Autodesk Inventor part; units mm, degrees
(part 2 of 2)
  spline S173 degree 2 poles (16.9034, -201.3098) (17.5444, -201.3098) (18.2669, -201.9878) (18.2669, -202.5658) knots 0 0 0 1 2 2 2
  spline S174 degree 2 poles (18.2669, -202.5658) (18.2669, -202.8363) (18.1409, -203.2883) (18.0297, -203.481) knots 0 0 0 1 2 2 2
  spline S175 degree 2 poles (18.0297, -203.481) (17.9186, -203.681) (17.5963, -204.0738) (17.4184, -204.2627) knots 0 0 0 1 2 2 2
  spline S176 degree 2 poles (17.4184, -204.2627) (17.1294, -204.5777) (16.4218, -205.252) (16.2106, -205.4483) knots 0 0 0 1 2 2 2
  line L141 (16.2106, -205.4483) -> (18.4558, -205.4483)
  line L142 (18.4558, -205.4483) -> (18.4558, -205.9782)
  line L143 (20.9678, -201.2024) -> (19.1783, -206.9711)
  line L144 (19.1783, -206.9711) -> (18.6596, -206.9711)
  line L145 (18.6596, -206.9711) -> (20.4417, -201.2024)
  line L146 (20.4417, -201.2024) -> (20.9678, -201.2024)
  line L147 (24.2912, -205.9782) -> (21.4717, -205.9782)
  line L148 (21.4717, -205.9782) -> (21.4717, -205.3298)
  spline S177 degree 2 poles (21.4717, -205.3298) (21.7755, -205.0445) (22.3165, -204.5147) (22.5758, -204.2294) knots 0 0 0 1 2 2 2
  spline S178 degree 2 poles (22.5758, -204.2294) (23.0982, -203.6551) (23.4798, -202.966) (23.4798, -202.5992) knots 0 0 0 1 2 2 2
  spline S179 degree 2 poles (23.4798, -202.5992) (23.4798, -202.4065) (23.3613, -202.1175) (23.2538, -202.0249) knots 0 0 0 1 2 2 2
  spline S180 degree 2 poles (23.2538, -202.0249) (23.1464, -201.9323) (22.8648, -201.8396) (22.6944, -201.8396) knots 0 0 0 1 2 2 2
  spline S181 degree 2 poles (22.6944, -201.8396) (22.5314, -201.8396) (22.1979, -201.9211) (22.046, -201.9841) knots 0 0 0 1 2 2 2
  spline S182 degree 2 poles (22.046, -201.9841) (21.9163, -202.036) (21.6755, -202.1842) (21.6014, -202.2361) knots 0 0 0 1 2 2 2
  line L149 (21.6014, -202.2361) -> (21.568, -202.2361)
  line L150 (21.568, -202.2361) -> (21.568, -201.584)
  spline S183 degree 2 poles (21.568, -201.584) (21.757, -201.4914) (22.435, -201.3098) (22.7388, -201.3098) knots 0 0 0 1 2 2 2
  spline S184 degree 2 poles (22.7388, -201.3098) (23.3798, -201.3098) (24.1023, -201.9878) (24.1023, -202.5658) knots 0 0 0 1 2 2 2
  spline S185 degree 2 poles (24.1023, -202.5658) (24.1023, -202.8363) (23.9763, -203.2883) (23.8652, -203.481) knots 0 0 0 1 2 2 2
  spline S186 degree 2 poles (23.8652, -203.481) (23.754, -203.681) (23.4317, -204.0738) (23.2538, -204.2627) knots 0 0 0 1 2 2 2
  spline S187 degree 2 poles (23.2538, -204.2627) (22.9648, -204.5777) (22.2572, -205.252) (22.046, -205.4483) knots 0 0 0 1 2 2 2
  line L151 (22.046, -205.4483) -> (24.2912, -205.4483)
  line L152 (24.2912, -205.4483) -> (24.2912, -205.9782)
  spline S188 degree 2 poles (27.748, -203.6922) (27.748, -204.9222) (27.033, -206.0745) (26.2882, -206.0745) knots 0 0 0 1 2 2 2
  spline S189 degree 2 poles (26.2882, -206.0745) (25.5324, -206.0745) (24.8248, -204.9) (24.8248, -203.6959) knots 0 0 0 1 2 2 2
  spline S190 degree 2 poles (24.8248, -203.6959) (24.8248, -202.4584) (25.5398, -201.3135) (26.2882, -201.3135) knots 0 0 0 1 2 2 2
  spline S191 degree 2 poles (26.2882, -201.3135) (27.0404, -201.3135) (27.748, -202.4991) (27.748, -203.6922) knots 0 0 0 1 2 2 2
  spline S192 degree 2 poles (26.9626, -205.0852) (27.0515, -204.8592) (27.1256, -204.1627) (27.1256, -203.6922) knots 0 0 0 1 2 2 2
  spline S193 degree 2 poles (27.1256, -203.6922) (27.1256, -203.2216) (27.0515, -202.5288) (26.9589, -202.2954) knots 0 0 0 1 2 2 2
  spline S194 degree 2 poles (26.9589, -202.2954) (26.8662, -202.0619) (26.5439, -201.8211) (26.2882, -201.8211) knots 0 0 0 1 2 2 2
  spline S195 degree 2 poles (26.2882, -201.8211) (26.0326, -201.8211) (25.7029, -202.0619) (25.6065, -202.3028) knots 0 0 0 1 2 2 2
  spline S196 degree 2 poles (25.6065, -202.3028) (25.5139, -202.5362) (25.4472, -203.2475) (25.4472, -203.6959) knots 0 0 0 1 2 2 2
  spline S197 degree 2 poles (25.4472, -203.6959) (25.4472, -204.1775) (25.5065, -204.8222) (25.6028, -205.0741) knots 0 0 0 1 2 2 2
  spline S198 degree 2 poles (25.6028, -205.0741) (25.6917, -205.3112) (26.0215, -205.5669) (26.2882, -205.5669) knots 0 0 0 1 2 2 2
  spline S199 degree 2 poles (26.2882, -205.5669) (26.5402, -205.5669) (26.8699, -205.3261) (26.9626, -205.0852) knots 0 0 0 1 2 2 2
  line L153 (31.1529, -205.9782) -> (28.3334, -205.9782)
  line L154 (28.3334, -205.9782) -> (28.3334, -205.3298)
  spline S200 degree 2 poles (28.3334, -205.3298) (28.6372, -205.0445) (29.1782, -204.5147) (29.4375, -204.2294) knots 0 0 0 1 2 2 2
  spline S201 degree 2 poles (29.4375, -204.2294) (29.9599, -203.6551) (30.3415, -202.966) (30.3415, -202.5992) knots 0 0 0 1 2 2 2
  spline S202 degree 2 poles (30.3415, -202.5992) (30.3415, -202.4065) (30.223, -202.1175) (30.1155, -202.0249) knots 0 0 0 1 2 2 2
  spline S203 degree 2 poles (30.1155, -202.0249) (30.0081, -201.9323) (29.7265, -201.8396) (29.5561, -201.8396) knots 0 0 0 1 2 2 2
  spline S204 degree 2 poles (29.5561, -201.8396) (29.3931, -201.8396) (29.0596, -201.9211) (28.9077, -201.9841) knots 0 0 0 1 2 2 2
  spline S205 degree 2 poles (28.9077, -201.9841) (28.778, -202.036) (28.5372, -202.1842) (28.4631, -202.2361) knots 0 0 0 1 2 2 2
  line L155 (28.4631, -202.2361) -> (28.4297, -202.2361)
  line L156 (28.4297, -202.2361) -> (28.4297, -201.584)
  spline S206 degree 2 poles (28.4297, -201.584) (28.6187, -201.4914) (29.2967, -201.3098) (29.6005, -201.3098) knots 0 0 0 1 2 2 2
  spline S207 degree 2 poles (29.6005, -201.3098) (30.2415, -201.3098) (30.964, -201.9878) (30.964, -202.5658) knots 0 0 0 1 2 2 2
  spline S208 degree 2 poles (30.964, -202.5658) (30.964, -202.8363) (30.838, -203.2883) (30.7269, -203.481) knots 0 0 0 1 2 2 2
  spline S209 degree 2 poles (30.7269, -203.481) (30.6157, -203.681) (30.2934, -204.0738) (30.1155, -204.2627) knots 0 0 0 1 2 2 2
  spline S210 degree 2 poles (30.1155, -204.2627) (29.8265, -204.5777) (29.1189, -205.252) (28.9077, -205.4483) knots 0 0 0 1 2 2 2
  line L157 (28.9077, -205.4483) -> (31.1529, -205.4483)
  line L158 (31.1529, -205.4483) -> (31.1529, -205.9782)
  spline S211 degree 2 poles (34.6542, -204.4961) (34.6542, -204.8481) (34.4208, -205.4446) (34.2244, -205.6447) knots 0 0 0 1 2 2 2
  spline S212 degree 2 poles (34.2244, -205.6447) (34.0206, -205.8559) (33.5093, -206.0745) (33.2018, -206.0745) knots 0 0 0 1 2 2 2
  spline S213 degree 2 poles (33.2018, -206.0745) (32.8943, -206.0745) (32.3867, -205.867) (32.1941, -205.6595) knots 0 0 0 1 2 2 2
  spline S214 degree 2 poles (32.1941, -205.6595) (31.9569, -205.4113) (31.6902, -204.5777) (31.6902, -203.97) knots 0 0 0 1 2 2 2
  spline S215 degree 2 poles (31.6902, -203.97) (31.6902, -203.3735) (31.9347, -202.4139) (32.1903, -202.0582) knots 0 0 0 1 2 2 2
  spline S216 degree 2 poles (32.1903, -202.0582) (32.4386, -201.71) (33.2241, -201.3209) (33.739, -201.3209) knots 0 0 0 1 2 2 2
  spline S217 degree 2 poles (33.739, -201.3209) (33.891, -201.3209) (34.1577, -201.3506) (34.2578, -201.3839) knots 0 0 0 1 2 2 2
  line L159 (34.2578, -201.3839) -> (34.2578, -201.973)
  line L160 (34.2578, -201.973) -> (34.2318, -201.973)
  spline S218 degree 2 poles (34.2318, -201.973) (34.1466, -201.9286) (33.8354, -201.8508) (33.6575, -201.8508) knots 0 0 0 1 2 2 2
  spline S219 degree 2 poles (33.6575, -201.8508) (33.087, -201.8508) (32.3867, -202.6214) (32.32, -203.3772) knots 0 0 0 1 2 2 2
  spline S220 degree 2 poles (32.32, -203.3772) (32.5386, -203.2253) (32.998, -203.0586) (33.2722, -203.0586) knots 0 0 0 1 2 2 2
  spline S221 degree 2 poles (33.2722, -203.0586) (33.539, -203.0586) (33.9391, -203.166) (34.1577, -203.3291) knots 0 0 0 1 2 2 2
  spline S222 degree 2 poles (34.1577, -203.3291) (34.4097, -203.518) (34.6542, -204.1034) (34.6542, -204.4961) knots 0 0 0 1 2 2 2
  spline S223 degree 2 poles (34.0317, -204.5221) (34.0317, -204.2405) (33.8835, -203.8589) (33.7205, -203.7255) knots 0 0 0 1 2 2 2
  spline S224 degree 2 poles (33.7205, -203.7255) (33.5983, -203.6292) (33.2944, -203.5662) (33.1351, -203.5662) knots 0 0 0 1 2 2 2
  spline S225 degree 2 poles (33.1351, -203.5662) (32.9202, -203.5662) (32.5164, -203.6959) (32.32, -203.8181) knots 0 0 0 1 2 2 2
  spline S226 degree 2 poles (32.32, -203.8181) (32.3163, -203.8848) (32.3089, -204.0108) (32.3089, -204.1071) knots 0 0 0 1 2 2 2
  spline S227 degree 2 poles (32.3089, -204.1071) (32.3089, -204.5814) (32.4942, -205.163) (32.635, -205.315) knots 0 0 0 1 2 2 2
  spline S228 degree 2 poles (32.635, -205.315) (32.7646, -205.4594) (33.0462, -205.5743) (33.2055, -205.5743) knots 0 0 0 1 2 2 2
  spline S229 degree 2 poles (33.2055, -205.5743) (33.576, -205.5743) (34.0317, -205.0482) (34.0317, -204.5221) knots 0 0 0 1 2 2 2
  point P0 (0, 0)
  constraints: 2 other
emboss "Emboss1" sketch "Sketch14" operation cut depth 2.54 direction (-1, 0, 0)
sketch "Sketch16" plane through (5.08, 0, 0) normal (1, 0, 0) x (0, 0, -1)
  line L0 (-45.5467, -73.9362) -> (38.2733, -73.9362)
  line L1 (38.2733, -73.9362) -> (38.2733, -77.7462)
  line L2 (38.2733, -77.7462) -> (-45.5467, -77.7462)
  line L3 (-45.5467, -77.7462) -> (-45.5467, -73.9362)
  line L4 (38.9083, -211.0962) -> (-46.1817, -211.0962) projected
  line L5 (42.0833, 28.0448) -> (42.0833, -207.9212) projected
  line L6 (-49.3567, -207.9212) -> (-49.3567, 28.0448) projected
  point P0 (0, 0)
  point P1 (38.9083, -223.7962)
  point P2 (42.0833, -220.6212)
  point P3 (38.2733, -75.8412)
  point P4 (-45.5467, -75.8412)
  dimension "d195" = 3.81
  dimension "d692" = 137.16
  dimension "d796" = 3.81
  dimension "d797" = 3.81
  constraints: 8 end point, 2 midpoint, 2 parallel, 1 horizontal, 1 perpendicular, 1 other
  measures "d195" distance between parallel lines of L0 L2
  measures "d796" distance from line of L5 point (38.273, -75.841)
  measures "d797" distance from line of L6 point (-45.547, -75.841)
extrude "Extrusion13" add sketch "Sketch16" along normal blind 5.08
sketch "Sketch17" plane through (24.13, 33.2264, 43.0067) normal (0, 1, 0) x (1, 0, 0)
  line L0 (-8.128, 57.15) -> (0, 57.15) projected
  line L1 (-0.0061, 57.15) -> (0.0392, 57.15)
  line L2 (0, 87.0966) -> (0, -8.3566) projected
  line L3 (0, 35.5801) -> (0, 35.5243)
  line L4 (5, -5.1816) -> (5, 83.9216) projected
  line L5 (0, 57.15) -> (5, 57.15)
  line L6 (5, 57.15) -> (5, 0)
  line L7 (5, 0) -> (0, 0)
  line L8 (0, 0) -> (0, 57.15)
  line L9 (0, 0) -> (-8.128, 0) projected
  point P0 (-24.13, 43.0067)
  point P1 (5, -23.8506)
  point P2 (5, 69.0626)
  point P3 (0, 0)
  point P4 (5, 57.15)
  point P5 (2.5, 0)
  point P6 (2.5, 57.15)
  dimension "d689" = 57.15
  dimension "d1196" = 0
  constraints: 12 end point, 4 point on line, 2 horizontal, 2 midpoint, 2 parallel, 1 perpendicular
  measures "d689" distance of point (2.5, 0) point (2.5, 57.15)
  measures "d1196" distance between parallel lines of L7 L9
extrude "Extrusion14" cut sketch "Sketch17" against normal blind 2.0066
sketch "Sketch18" plane through (0, 0, 0) normal (-1, 0, 0) x (0, 0, 1)
  arc A0 (48.3408, 33.2227) -> (51.3596, 30.2039) centre (50.6267, 32.4898) ccw projected
  circle A1 centre (50.6267, 32.4898) radius 4.5085
  arc A2 (-41.0674, 33.2227) -> (-44.0862, 30.2039) centre (-43.3533, 32.4898) ccw projected
  circle A3 centre (-43.3533, 32.4898) radius 4.5085
  arc A4 (-44.0862, -210.0804) -> (-41.0674, -213.0992) centre (-43.3533, -212.3662) ccw projected
  circle A5 centre (-43.3533, -212.3662) radius 4.5085
  arc A6 (48.3408, -213.0992) -> (51.3596, -210.0804) centre (50.6267, -212.3662) ccw projected
  circle A7 centre (50.6267, -212.3662) radius 4.5085
  point P0 (0, 0)
  point P1 (-44.0899, -210.0815)
  point P2 (-44.0899, -214.6509)
  point P3 (48.8233, -214.6509)
  point P4 (48.8233, -210.0815)
  point P5 (-41.0686, 33.2264)
  point P6 (-41.0686, -213.1028)
  dimension "d209" = 9.017
  dimension "d210" = 9.017
  dimension "d211" = 9.017
  dimension "d212" = 9.017
  constraints: 4 centre point, 4 coincident
  measures "d209" diameter of A1
  measures "d210" diameter of A3
  measures "d211" diameter of A5
  measures "d212" diameter of A7
extrude "Extrusion15" [suppressed]
sketch "Sketch19" plane through (24.13, -51.5842, -44.0899) normal (0, 0, -1) x (-1, 0, 0)
  line L0 (7.62, 0) -> (0, 0) projected
  line L1 (-5, 79.629) -> (-5, -156.337) projected
  line L2 (0, 0) -> (-5, 0)
  line L3 (-5, 0) -> (-5, 8.001)
  line L4 (-5, 8.001) -> (0, 8.001)
  line L5 (0, 8.001) -> (0, 0)
  point P0 (24.13, 51.5842)
  point P1 (-5, -156.337)
  dimension "d216" = 5
  dimension "d219" = 8.001
  constraints: 8 end point, 2 parallel, 1 horizontal, 1 perpendicular, 1 point on line
  measures "d216" distance between parallel lines of L1 L5
  measures "d219" distance between parallel lines of L2 L4
extrude "Extrusion16" cut sketch "Sketch19" against normal blind 24.13
sketch "Sketch20" plane through (0, 0, 0) normal (-1, 0, 0) x (0, 0, 1)
  line L0 (-45.1249, 28.9592) -> (-41.5943, 28.9592)
  line L1 (-45.1249, 36.0204) -> (-41.5943, 36.0204)
  line L2 (-45.1249, 28.9592) -> (-47.1633, 32.4898)
  line L3 (-45.1249, 36.0204) -> (-47.1633, 32.4898)
  line L4 (-41.5943, 28.9592) -> (-39.5559, 32.4898)
  line L5 (-41.5943, 36.0204) -> (-39.5559, 32.4898)
  line L6 (-45.1249, -215.8968) -> (-41.5943, -215.8968)
  line L7 (-45.1249, -208.8356) -> (-41.5943, -208.8356)
  line L8 (-45.1249, -215.8968) -> (-47.1633, -212.3662)
  line L9 (-45.1249, -208.8356) -> (-47.1633, -212.3662)
  line L10 (-41.5943, -215.8968) -> (-39.5559, -212.3662)
  line L11 (-41.5943, -208.8356) -> (-39.5559, -212.3662)
  line L12 (48.8551, 28.9592) -> (52.3857, 28.9592)
  line L13 (48.8551, 36.0204) -> (52.3857, 36.0204)
  line L14 (48.8551, 28.9592) -> (46.8167, 32.4898)
  line L15 (48.8551, 36.0204) -> (46.8167, 32.4898)
  line L16 (52.3857, 28.9592) -> (54.4241, 32.4898)
  line L17 (52.3857, 36.0204) -> (54.4241, 32.4898)
  line L18 (48.8551, -215.8968) -> (52.3857, -215.8968)
  line L19 (48.8551, -208.8356) -> (52.3857, -208.8356)
  line L20 (48.8551, -215.8968) -> (46.8167, -212.3662)
  line L21 (48.8551, -208.8356) -> (46.8167, -212.3662)
  line L22 (52.3857, -215.8968) -> (54.4241, -212.3662)
  line L23 (52.3857, -208.8356) -> (54.4241, -212.3662)
  line L24 (-40.0449, -67.5608) -> (-36.5143, -67.5608)
  line L25 (-40.0449, -60.4996) -> (-36.5143, -60.4996)
  line L26 (-40.0449, -67.5608) -> (-42.0833, -64.0302)
  line L27 (-40.0449, -60.4996) -> (-42.0833, -64.0302)
  line L28 (-36.5143, -67.5608) -> (-34.4759, -64.0302)
  line L29 (-36.5143, -60.4996) -> (-34.4759, -64.0302)
  line L30 (43.7751, -67.5608) -> (47.3057, -67.5608)
  line L31 (43.7751, -60.4996) -> (47.3057, -60.4996)
  line L32 (43.7751, -67.5608) -> (41.7367, -64.0302)
  line L33 (43.7751, -60.4996) -> (41.7367, -64.0302)
  line L34 (47.3057, -67.5608) -> (49.3441, -64.0302)
  line L35 (47.3057, -60.4996) -> (49.3441, -64.0302)
  point P0 (0, 0)
  point P1 (-16.6833, 31.2198)
  point P2 (-43.3596, 28.9592)
  point P3 (-43.3533, 32.4898)
  point P4 (-43.3596, -215.8968)
  point P5 (50.6204, 28.9592)
  point P6 (50.6204, -215.8968)
  point P7 (-38.2796, -67.5608)
  point P8 (45.5404, -67.5608)
  dimension "d963" = 7.0612
  dimension "d964" = 120
  dimension "d965" = 120
  dimension "d966" = 120
  dimension "d967" = 120
  dimension "d968" = 3.5306
  dimension "d969" = 3.5306
  dimension "d970" = 3.5306
  dimension "d971" = 3.5306
  dimension "d972" = 3.5306
  dimension "d973" = 3.5306
  dimension "d974" = 0
  dimension "d975" = 7.6074
  dimension "d1031" = 7.0612
  dimension "d1032" = 120
  dimension "d1033" = 120
  dimension "d1034" = 120
  dimension "d1035" = 120
  dimension "d1036" = 3.5306
  dimension "d1037" = 3.5306
  dimension "d1038" = 3.5306
  dimension "d1039" = 3.5306
  dimension "d1040" = 3.5306
  dimension "d1041" = 3.5306
  dimension "d1042" = 0
  dimension "d1043" = 7.6074
  dimension "d1082" = 7.0612
  dimension "d1083" = 120
  dimension "d1084" = 120
  dimension "d1085" = 120
  dimension "d1086" = 120
  dimension "d1087" = 3.5306
  dimension "d1088" = 3.5306
  dimension "d1089" = 3.5306
  dimension "d1090" = 3.5306
  dimension "d1091" = 3.5306
  dimension "d1092" = 3.5306
  dimension "d1093" = 0
  dimension "d1094" = 7.6074
  dimension "d1116" = 7.0612
  dimension "d1117" = 120
  dimension "d1118" = 120
  dimension "d1119" = 120
  dimension "d1120" = 120
  dimension "d1121" = 3.5306
  dimension "d1122" = 3.5306
  dimension "d1123" = 3.5306
  dimension "d1124" = 3.5306
  dimension "d1125" = 3.5306
  dimension "d1126" = 3.5306
  dimension "d1127" = 0
  dimension "d1128" = 7.6074
  dimension "d1160" = 7.0612
  dimension "d1161" = 120
  dimension "d1162" = 120
  dimension "d1163" = 120
  dimension "d1164" = 120
  dimension "d1165" = 3.5306
  dimension "d1166" = 3.5306
  dimension "d1167" = 3.5306
  dimension "d1168" = 3.5306
  dimension "d1169" = 3.5306
  dimension "d1170" = 3.5306
  dimension "d1171" = 0
  constraints: 72 end point, 12 horizontal, 6 midpoint
  measures "d963" distance from line of point (-43.36, 28.959) L1
  measures "d964" angle of L0 L2
  measures "d965" angle of L1 L3
  measures "d966" angle of L4 L0
  measures "d967" angle of L5 L1
  measures "d968" distance of L0.start L4.start
  measures "d969" distance of L1.start L5.start
  measures "d970" vertical distance of L1.start L3.end
  measures "d971" vertical distance of L0.start L2.end
  measures "d972" vertical distance of L5.start L5.end
  measures "d973" vertical distance of L4.start L4.end
  measures "d974" horizontal distance of L0.start L1.start
  measures "d975" distance of L4.end L2.end
  measures "d1031" distance from line of point (-43.36, -215.897) L7
  measures "d1032" angle of L6 L8
  measures "d1033" angle of L7 L9
  measures "d1034" angle of L10 L6
  measures "d1035" angle of L11 L7
  measures "d1036" distance of L6.start L10.start
  measures "d1037" distance of L7.start L11.start
  measures "d1038" vertical distance of L7.start L9.end
  measures "d1039" vertical distance of L6.start L8.end
  measures "d1040" vertical distance of L11.start L11.end
  measures "d1041" vertical distance of L10.start L10.end
  measures "d1042" horizontal distance of L6.start L7.start
  measures "d1043" distance of L10.end L8.end
  measures "d1082" distance from line of point (50.62, 28.959) L13
  measures "d1083" angle of L12 L14
  measures "d1084" angle of L13 L15
  measures "d1085" angle of L16 L12
  measures "d1086" angle of L17 L13
  measures "d1087" distance of L12.start L16.start
  measures "d1088" distance of L15.start L17.start
  measures "d1089" vertical distance of L15.start L15.end
  measures "d1090" vertical distance of L12.start L14.end
  measures "d1091" vertical distance of L17.start L17.end
  measures "d1092" vertical distance of L16.start L16.end
  measures "d1093" horizontal distance of L12.start L15.start
  measures "d1094" distance of L16.end L14.end
  measures "d1116" distance from line of point (50.62, -215.897) L19
  measures "d1117" angle of L18 L20
  measures "d1118" angle of L19 L21
  measures "d1119" angle of L22 L18
  measures "d1120" angle of L23 L19
  measures "d1121" distance of L18.start L22.start
  measures "d1122" distance of L21.start L23.start
  measures "d1123" vertical distance of L21.start L21.end
  measures "d1124" vertical distance of L18.start L20.end
  measures "d1125" vertical distance of L23.start L23.end
  measures "d1126" vertical distance of L22.start L22.end
  measures "d1127" horizontal distance of L18.start L21.start
  measures "d1128" distance of L22.end L20.end
  measures "d1160" distance from line of point (-38.28, -67.561) L25
  measures "d1161" angle of L24 L26
  measures "d1162" angle of L25 L27
  measures "d1163" angle of L28 L24
  measures "d1164" angle of L29 L25
  measures "d1165" distance of L24.start L28.start
  measures "d1166" distance of L25.start L29.start
  measures "d1167" vertical distance of L25.start L27.end
  measures "d1168" vertical distance of L24.start L26.end
  measures "d1169" vertical distance of L29.start L29.end
  measures "d1170" vertical distance of L28.start L28.end
  measures "d1171" horizontal distance of L24.start L25.start
extrude "Extrusion18" cut sketch "Sketch20" against normal blind 4
sketch "Sketch21" plane through (5.08, 0, 0) normal (1, 0, 0) x (0, 0, -1)
  line L0 (-49.3567, -207.9212) -> (-49.3567, 28.0448) projected
  line L1 (42.0833, -69.6717) -> (42.0833, -83.8957)
  line L2 (44.0899, -209.9278) -> (44.0899, -51.5842) projected
  line L3 (-49.3567, -83.8422) -> (-49.3567, -69.6182)
  line L4 (-42.4987, -58.8939) -> (-42.4987, -69.23)
  line L5 (-44.2301, -72.0578) -> (-47.3797, -73.6657)
  line L6 (-48.7308, -74.9867) -> (-49.3567, -76.1476)
  line L7 (-44.2301, -56.0661) -> (-47.3797, -54.4582)
  line L8 (-48.7639, -53.074) -> (-49.3567, -51.9128)
  arc A0 (-47.3797, -73.6657) -> (-48.7308, -74.9867) centre (-45.9361, -76.4935) ccw
  arc A1 (-44.2301, -72.0578) -> (-42.4987, -69.23) centre (-45.6737, -69.23) ccw
  arc A2 (-42.4987, -58.8939) -> (-44.2301, -56.0661) centre (-45.6737, -58.8939) ccw
  arc A3 (-48.7639, -53.074) -> (-47.3797, -54.4582) centre (-45.9361, -51.6304) ccw
  line L9 (-49.3567, -51.9128) -> (-49.3567, -76.1476)
  arc A4 (-47.9472, -64.0302) -> (-47.9472, -64.0302) centre (-45.5467, -64.0302) ccw projected
  circle A5 centre (-45.5467, -64.0302) radius 2.4005
  line L10 (35.2253, -69.1835) -> (35.2253, -58.8478)
  line L11 (36.9569, -56.0198) -> (40.1065, -54.4123)
  line L12 (41.4675, -53.0729) -> (42.0833, -51.9128)
  line L13 (36.9569, -72.0115) -> (40.1065, -73.619)
  line L14 (41.4675, -74.9584) -> (42.0833, -76.1184)
  arc A6 (41.4675, -74.9584) -> (40.1065, -73.619) centre (38.6631, -76.447) ccw
  arc A7 (35.2253, -69.1835) -> (36.9569, -72.0115) centre (38.4003, -69.1835) ccw
  arc A8 (40.1065, -54.4123) -> (41.4675, -53.0729) centre (38.6631, -51.5843) ccw
  arc A9 (36.9569, -56.0198) -> (35.2253, -58.8478) centre (38.4003, -58.8478) ccw
  line L15 (42.0833, -51.9128) -> (42.0833, -76.1184)
  line L16 (42.0833, -51.9128) -> (42.0833, -76.1184)
  circle A10 centre (38.2733, -64.0302) radius 2.4005 projected
  line L17 (42.0833, -51.5842) -> (42.0833, -43.5842) projected
  circle A11 centre (53.1966, -64.0156) radius 2.0413
  point P0 (0, 0)
  point P1 (-43.0067, -58.9502)
  point P2 (-48.2611, -74.1156)
  point P3 (-48.2961, -53.9904)
  point P4 (-43.0067, -74.3297)
  point P5 (-40.8318, -77.7462)
  point P6 (40.9982, -53.9572)
  dimension "d785" = 6.858
  dimension "d786" = 117.044
  dimension "d787" = 117.044
  dimension "d792" = 2.032
  dimension "d793" = 3.175
  dimension "d794" = 3.1496
  dimension "d795" = 3.1496
  dimension "d917" = 24.2348
  dimension "d1137" = 4.801
  dimension "d1144" = 145
  dimension "d1145" = 145
  dimension "d1146" = 117.04
  dimension "d1147" = 117.04
  dimension "d1148" = 3.175
  dimension "d1149" = 3.175
  dimension "d1150" = 3.1496
  dimension "d1151" = 2.0443
  dimension "d1152" = 3.1496
  dimension "d1153" = 24.2056
  dimension "d1155" = 0
  dimension "d1156" = 12.1028
  dimension "d1157" = 14.9233
  dimension "d1158" = 12.1174
  dimension "d1159" = 12.1174
  constraints: 30 end point, 16 point on circle, 16 tangent, 10 centre point, 9 point on line, 5 equal radius, 2 vertical, 1 coincident, 1 collinear, 1 parallel, 1 perpendicular
  measures "d785" distance between parallel lines of L0 L4
  measures "d786" angle of L5 L4
  measures "d787" angle of L7 L4
  measures "d792" vertical distance of point (-48.261, -74.116) L6.end
  measures "d793" radius of A0
  measures "d794" horizontal distance of L5.start L5.end
  measures "d795" horizontal distance of L7.start L7.end
  measures "d917" distance of L6.end L8.end
  measures "d1137" diameter of A5
  measures "d1144" angle of L11 L12
  measures "d1145" angle of L14 L13
  measures "d1146" angle of L13 L10
  measures "d1147" angle of L10 L11
  measures "d1148" radius of A6
  measures "d1149" radius of A8
  measures "d1150" horizontal distance of L11.start L11.end
  measures "d1151" vertical distance of L12.end point (40.998, -53.957)
  measures "d1152" horizontal distance of L13.start L13.end
  measures "d1153" distance of L14.end L12.end
  measures "d1155" distance between parallel lines of L17 L15
  measures "d1156" vertical distance of L12.end A11.centre
  measures "d1157" distance of A10.centre A11.centre
  measures "d1158" vertical distance of A4.centre L8.end
  measures "d1159" vertical distance of A10.centre L12.end
extrude "Extrusion19" add sketch "Sketch21" along normal blind 22.86 contours L0 L8 A3 L7 A2 L4 A1 L5 A0 L6 | L1 L14 A6 L13 A7 L10 A9 L11 A8 L12 L15
sketch "Sketch22" plane through (16.08, -230.1462, -3.2973) normal (0, -1, 0) x (1, 0, 0)
  circle A0 centre (2.2292, -12.1283) radius 2.032
  line L0 (-16.08, -45.136) -> (8.05, -45.136) projected
  circle A1 centre (10.002, -12.1283) radius 2.032
  line L1 (13.05, 48.9456) -> (13.05, -37.6176) projected
  point P0 (-16.08, 3.2973)
  dimension "d445" = 4.064
  dimension "d446" = 33.0076
  dimension "d449" = 4.064
  dimension "d450" = 3.048
  constraints: 2 centre point
  measures "d445" diameter of A0
  measures "d446" distance from line of L0 A0.centre
  measures "d449" diameter of A1
  measures "d450" distance from line of L1 A1.centre
extrude "Extrusion20" [suppressed]
fillet "Fillet6" radius 0.508 8 edges at (20.32, -51.5842, -48.4333) (20.32, -43.5842, -48.4333) (16.51, -47.5842, -48.4333) (20.066, 37.5698, -14.1433) (16.002, 37.5698, 14.4317) (20.066, 37.5698, 43.0067) (26.63, 33.2264, 43.0067) (26.63, -43.5832, -44.0899)
sketch "Sketch23" plane through (22.86, -225.8028, -3.2973) normal (0, -1, 0) x (1, 0, 0)
  line L0 (1.27, -37.6176) -> (1.27, 48.9456) projected
  line L1 (6.27, 48.9456) -> (6.27, -37.6176) projected
  line L2 (0, 10) -> (6.27, 10)
  line L3 (6.27, 10) -> (6.27, -0.0129)
  line L4 (6.27, -0.0129) -> (0, -0.0129)
  line L5 (0, -0.0129) -> (0, 10)
  point P0 (-22.86, 3.2973)
  point P1 (1.27, 48.9456)
  constraints: 8 end point, 2 parallel, 1 horizontal, 1 perpendicular, 1 point on line, 1 other
extrude "Extrusion21" [suppressed]
sketch "Sketch24" plane through (8.636, -223.7962, -3.2973) normal (0, 1, 0) x (1, 0, 0)
  circle A0 centre (9.652, -31.318) radius 4.445
  line L0 (-3.556, 35.611) -> (-3.556, -46.939) projected
  point P0 (-8.636, -3.2973)
  point P1 (15.494, -56.464)
  dimension "d673" = 25.146
  dimension "d674" = 13.208
  dimension "d677" = 8.89
  constraints: 1 centre point
  measures "d673" vertical distance of point (15.494, -56.464) A0.centre
  measures "d674" distance from line of L0 A0.centre
  measures "d677" diameter of A0
extrude "Extrusion22" [suppressed]
sketch "Sketch25" plane through (5.08, 0, 0) normal (1, 0, 0) x (0, 0, -1)
  line L0 (-49.3567, 15.9798) -> (20.6609, 15.9798)
  line L1 (11.7709, 3.2798) -> (-49.3567, 3.2798)
  line L2 (-49.3567, 3.2798) -> (-49.3567, 15.9798)
  circle A0 centre (-32.8467, 9.6298) radius 2.4005 projected
  circle A1 centre (4.1509, 9.6298) radius 2.4005 projected
  circle A2 centre (-14.3479, 9.6298) radius 2.4005 projected
  line L3 (-49.3567, -207.9212) -> (-49.3567, 28.0448) projected
  line L4 (42.0833, 28.0448) -> (42.0833, -43.5832) projected
  line L5 (20.6609, 15.9798) -> (42.0833, 15.9798)
  line L6 (42.0833, 15.9798) -> (42.0833, 3.2798)
  line L7 (42.0833, 3.2798) -> (11.7709, 3.2798)
  point P0 (0, 0)
  point P1 (-14.3479, 15.9798)
  point P2 (-46.8167, -36.8286)
  point P3 (-49.3567, 28.0448)
  point P4 (42.0833, -36.6918)
  dimension "d680" = 6.35
  dimension "d681" = 6.35
  dimension "d682" = 0
  dimension "d685" = 0
  dimension "d686" = 12.7
  constraints: 12 end point, 2 horizontal, 2 parallel, 1 midpoint, 1 perpendicular, 1 other
  measures "d680" distance of point (-14.348, 15.98) A2.centre
  measures "d681" distance from line of L1 A2.centre
  measures "d682" horizontal extent of L2
  measures "d685" distance between parallel lines of L4 L6
  measures "d686" distance between parallel lines of L7 L5
extrude "Extrusion23" add sketch "Sketch25" along normal blind 10.16
sketch "Sketch26" plane through (0, -217.4462, -45.2583) normal (0, -1, 0) x (1, 0, 0)
  line L0 (29.13, 88.265) -> (10.3097, 88.265)
  line L1 (10.3097, 9.525) -> (29.13, 9.525)
  line L2 (29.13, 9.525) -> (29.13, 88.265)
  line L3 (0, -3.175) -> (24.13, -3.175) projected
  line L4 (24.13, 100.965) -> (0, 100.965) projected
  line L5 (29.13, 93.4466) -> (29.13, 4.3434) projected
  line L6 (8.7811, 88.265) -> (8.7811, 85.0428)
  line L7 (10.3097, 88.265) -> (8.7811, 88.265)
  line L8 (8.7811, 88.265) -> (8.7811, 9.525)
  line L9 (10.3097, 9.525) -> (8.7811, 9.525)
  point P0 (0, 45.2583)
  point P1 (29.13, 51.961)
  dimension "d832" = 12.7
  dimension "d833" = 12.7
  dimension "d837" = 0
  constraints: 14 end point, 2 horizontal, 2 perpendicular, 1 parallel, 1 vertical
  measures "d832" distance between parallel lines of L3 L1
  measures "d833" distance between parallel lines of L4 L0
  measures "d837" distance between parallel lines of L5 L2
extrude "Extrusion24" cut sketch "Sketch26" against normal blind 7.62
fillet "Fillet7" radius 0.762 4 edges at (17.2199, -217.4462, 43.0067) (9.5454, -217.4462, 43.0067) (17.2199, -217.4462, -35.7333) (9.5454, -217.4462, -35.7333)
body "Solid1"
